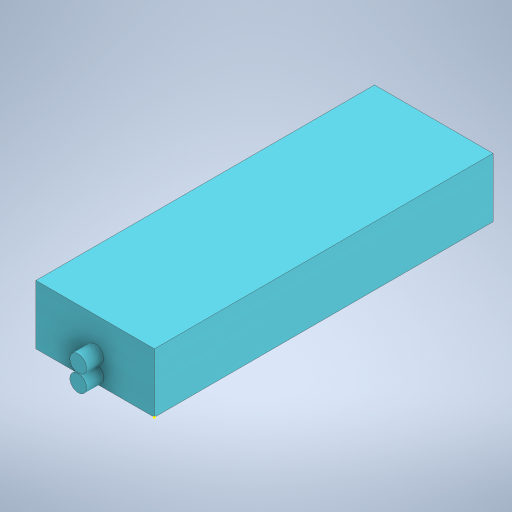
# Autodesk Inventor part: water tank mm
Saved by Autodesk Inventor 2024 (Build 280153000, 153)
## iProperties
Created: 2024-02-04
Part Number: water tank mm
Material: Generic
Document SubType Name: Modeling
Designer: RAHUL
Density: 1 g/cm^3
Appearance: Default
Author: RAHUL
Autodesk Inventor part; units mm, degrees
ref_plane "YZ Plane" through (0, 0, 0) normal (1, 0, 0) x (0, 1, 0)
ref_plane "XZ Plane" through (0, 0, 0) normal (0, 1, 0) x (-1, 0, 0)
ref_plane "XY Plane" through (0, 0, 0) normal (0, 0, 1) x (1, 0, 0)
sketch "Sketch1" plane through (0, 0, 0) normal (0, 1, 0) x (-1, 0, 0)
  line L0 (0, 0) -> (70, 0)
  line L1 (70, 0) -> (70, -200)
  line L2 (70, -200) -> (0, -200)
  line L3 (0, -200) -> (0, 0)
  dimension "d0" = 70
  dimension "d1" = 200
  constraints: 8 end point, 2 parallel, 1 horizontal, 1 perpendicular
  measures "d0" distance of L1.end L2.end
  measures "d1" distance of L0.end L1.end
extrude "Extrusion1" add sketch "Sketch1" along normal blind 35
sketch "Sketch2" plane through (-70, 0, 0) normal (0, 0, 1) x (1, 0, 0)
  point P0 (70, 0)
sketch "Sketch3" plane through (-70, 0, 0) normal (0, 0, 1) x (1, 0, 0)
  circle A0 centre (35, 5) radius 5
  circle A1 centre (35, 15) radius 5
  line L0 (70, 0) -> (70, 35) projected
  line L1 (0, 0) -> (70, 0) projected
  point P0 (70, 17.5)
  dimension "d4" = 10
  dimension "d5" = 10
  dimension "d6" = 35
  dimension "d7" = 35
  dimension "d8" = 10
  dimension "d9" = 5
  constraints: 2 centre point, 1 midpoint
  measures "d4" diameter of A0
  measures "d5" diameter of A1
  measures "d6" distance from line of L0 A0.centre
  measures "d7" horizontal distance of point (70, 17.5) A1.centre
  measures "d8" distance of A0.centre A1.centre
  measures "d9" distance from line of L1 A0.centre
extrude "Extrusion2" add sketch "Sketch3" along normal blind 10 contours A0
sketch "Sketch4" plane through (-70, 35, 0) normal (0, 0, 1) x (1, 0, 0)
  circle A0 centre (35, -20) radius 5
  line L0 (35, -35) -> (70, -35) projected
  line L1 (70, -35) -> (70, 0) projected
  dimension "d12" = 10
  dimension "d13" = 15
  dimension "d14" = 35
  constraints: 1 centre point
  measures "d12" diameter of A0
  measures "d13" distance from line of L0 A0.centre
  measures "d14" distance from line of L1 A0.centre
extrude "Extrusion3" add sketch "Sketch4" along normal blind 10
body "Solid1"
